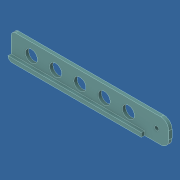
# Autodesk Inventor part: Lopez_LeftLeg
Saved by Autodesk Inventor 2018 (Build 220112000, 112)
## iProperties
Created: 2018-02-07
Part Number: Lopez_LeftLeg
Material: Polypropylene
Document SubType Name: Modeling
Designer: clopez06
Density: 0.899 g/cm^3
Appearance: Smooth - Ash
Mass: 2.77644 g
Surface Area: 36.2746 cm^2
Volume: 3.08837 cm^3
Author: clopez06
Autodesk Inventor part; units mm, degrees
ref_plane "YZ Plane" through (0, 0, 0) normal (1, 0, 0) x (0, 1, 0)
ref_plane "XZ Plane" through (0, 0, 0) normal (0, 1, 0) x (-1, 0, 0)
ref_plane "XY Plane" through (0, 0, 0) normal (0, 0, 1) x (1, 0, 0)
sketch "Sketch1" plane through (0, 0, 0) normal (0, 0, 1) x (1, 0, 0)
  point P0 (0, 0)
sketch "Sketch2" plane through (0, 0, 0) normal (0, 0, 1) x (1, 0, 0)
  line L0 (0, 0) -> (99.06, 0)
  line L1 (99.06, 0) -> (99.06, 15.24)
  line L2 (99.06, 15.24) -> (0, 15.24)
  line L3 (0, 15.24) -> (0, 0)
  dimension "d0" = 15.24
  dimension "d1" = 99.06
  constraints: 8 end point, 2 parallel, 1 horizontal, 1 perpendicular
  measures "d0" distance of L2.end L0.start
  measures "d1" distance of L1.end L2.end
extrude "Extrusion1" add sketch "Sketch2" along normal blind 2.032
sketch "Sketch3" plane through (0, 0, 2.032) normal (0, 0, 1) x (1, 0, 0)
  line L0 (0, 15.24) -> (0, 0) projected
  line L1 (0, 7.62) -> (99.06, 7.62)
  line L2 (99.06, 0) -> (99.06, 15.24) projected
  point P0 (12.7, 7.62)
  dimension "d14" = 12.7
  constraints: 2 end point, 2 midpoint, 1 point on line
  measures "d14" distance from line of L0 point (12.7, 7.62)
hole "Hole1" at (12.7, 7.62, 2.032) direction (0, 0, -1) diameter 7.62 end through all
pattern_linear "Rectangular Pattern1" count 5 spacing 15.24 along (1, 0, 0) of "Hole1"
sketch "Sketch4" plane through (0, 0, 2.032) normal (0, 0, 1) x (1, 0, 0)
  line L0 (99.06, 0) -> (99.06, 15.24) projected
  line L1 (99.06, 7.62) -> (91.44, 7.62)
  point P0 (0, 0)
  dimension "d15" = 7.62
  constraints: 2 end point, 1 horizontal, 1 midpoint
  measures "d15" distance of L1.start L1.end
hole "Hole2" at (91.44, 7.62, 2.032) direction (0, 0, -1) diameter 2.54 end through all
sketch "Sketch5" plane through (0, 0, 2.032) normal (0, 0, 1) x (1, 0, 0)
  line L0 (0, 0) -> (83.82, 0)
  line L1 (83.82, 0) -> (83.82, 2.54)
  line L2 (83.82, 2.54) -> (0, 2.54)
  line L3 (0, 2.54) -> (0, 0)
  dimension "d23" = 83.82
  dimension "d24" = 2.54
  constraints: 8 end point, 2 parallel, 1 horizontal, 1 perpendicular
  measures "d23" distance of L0.start L0.end
  measures "d24" distance of L2.end L0.start
extrude "Extrusion2" add sketch "Sketch5" along normal blind 2.032
fillet "Fillet1" radius 5.08 2 edges at (99.06, 15.24, 1.016) (99.06, 0, 1.016)
fillet "Fillet2" radius 2.54 2 edges at (0, 15.24, 1.016) (0, 0, 2.032)
equation "\"d15\" = 0.5 * d0"
body "Solid1"
